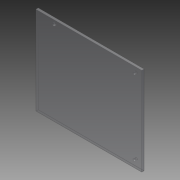
# Autodesk Inventor part: Wheel Shield 2
Saved by Autodesk Inventor 2014 SP1 (Build 180222100, 222)
## iProperties
Created: 2013-03-21
Part Number: Wheel Shield 2
Material: Polycarbonate, Clear
Document SubType Name: Modeling
Designer: actoennies
Mass: 73.638 g
Surface Area: 405.307 cm^2
Volume: 61.365 cm^3
Density: 1.2 g/cm^3
Appearance: Polycarbonate - Clear
Author: actoennies
Autodesk Inventor part; units mm, degrees
ref_plane "YZ Plane" through (0, 0, 0) normal (1, 0, 0) x (0, 1, 0)
ref_plane "XZ Plane" through (0, 0, 0) normal (0, 1, 0) x (-1, 0, 0)
ref_plane "XY Plane" through (0, 0, 0) normal (0, 0, 1) x (1, 0, 0)
sketch "Sketch1" plane through (0, 0, 0) normal (0, 0, 1) x (1, 0, 0)
  line L0 (0, 0) -> (0, 127)
  line L1 (0, 127) -> (152.4, 127)
  line L2 (152.4, 127) -> (152.4, 0)
  line L3 (152.4, 0) -> (0, 0)
  circle A0 centre (25.4, 120.65) radius 1.905
  line L4 (0, 120.65) -> (152.4, 120.65) construction
  circle A1 centre (141.2875, 117.475) radius 1.5875 projected
  circle A2 centre (141.2875, 9.525) radius 1.5875 projected
  dimension "d0" = 127
  dimension "d1" = 152.4
  dimension "d4" = 3.81
  dimension "d5" = 6.35
  dimension "d6" = 25.4
  constraints: 10 end point, 3 point on line, 2 perpendicular, 1 centre point, 1 horizontal, 1 parallel, 1 vertical
  measures "d0" distance of L0.start L0.end
  measures "d1" distance of L0.end L1.end
  measures "d4" diameter of A0
  measures "d5" distance between parallel lines of L1 L4
  measures "d6" distance from line of A0.centre L0
extrude "Extrusion1" add sketch "Sketch1" along normal blind 3.175
body "Solid1"
